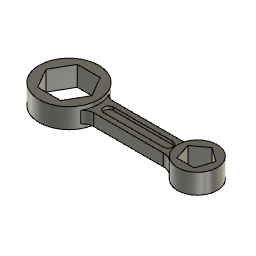
Exercise 2 (Autodesk Fusion 360 design; units mm, degrees)
Autodesk Fusion 360 part; units mm, degrees
sketch "Sketch1" plane through (0, 0, 0) normal (0, 0, 1) x (1, 0, 0)
  circle A0 centre (30, 30) radius 30
  line L0 (64.143, 40) -> (135, 40)
  line L1 (65, 20) -> (135, 20)
  circle A1 centre (159, 30.4309) radius 20
  line L2 (130, 34.8765) -> (70, 34.8765)
  arc A2 (70, 34.8765) -> (70, 25.1235) centre (70, 30) ccw
  line L3 (70, 25.1235) -> (130, 25.1235)
  arc A3 (130, 25.1235) -> (130, 34.8765) centre (130, 30) ccw
  line L4 (130, 30) -> (70, 30) construction
  line L5 (18.453, 50) -> (6.906, 30)
  line L6 (6.906, 30) -> (18.453, 10)
  line L7 (18.453, 10) -> (41.547, 10)
  line L8 (41.547, 10) -> (53.094, 30)
  line L9 (53.094, 30) -> (41.547, 50)
  line L10 (41.547, 50) -> (18.453, 50)
  line L11 (159, 45.216) -> (144.9385, 34.9998)
  line L12 (144.9385, 34.9998) -> (150.3095, 18.4695)
  line L13 (150.3095, 18.4695) -> (167.6905, 18.4695)
  line L14 (167.6905, 18.4695) -> (173.0615, 34.9998)
  line L15 (173.0615, 34.9998) -> (159, 45.216)
  arc A4 (56.3472, 44.3465) -> (64.143, 40) centre (64.143, 49.1644) ccw
  arc A5 (65, 20) -> (56.3472, 15.6535) centre (65, 9.2141) ccw
  arc A6 (145.5231, 15.6535) -> (135, 20) centre (135, 5.0883) ccw
  arc A7 (135, 40) -> (144.9303, 44.6452) centre (135, 52.937) ccw
  point P0 (30, 30)
  point P1 (159, 30.4309)
  point P2 (159, 45.216)
  point P3 (159, 30.4309)
  constraint horizontal L0
  constraint horizontal L1
  constraint tangent L2 A2
  constraint tangent A2 L3
  constraint parallel L2 L3
  constraint tangent L3 A3
  constraint tangent L2 A3
  constraint parallel L0 L4
  constraint coincident P0 A0.centre
  constraint coincident P3 P1
  constraint coincident P2 L11.start
  constraint tangent L0 A4
  constraint coincident A0 A4.start
  constraint tangent L1 A5
  constraint coincident A0 A5.end
  constraint tangent L1 A6
  constraint coincident A1 A6.start
  constraint tangent L0 A7
  constraint coincident A1 A7.end
extrude "Extrude1" add sketch "Sketch1" along normal mid plane 12 contours A0 L0 L1 A1 A4 A5 A6 A7
extrude "Extrude2" add sketch "Sketch1" along normal mid plane 20 contours A0 | A1 A6 A7
extrude "Extrude3" add sketch "Sketch1" along normal mid plane 6 contours L2 A2 L3 A3
